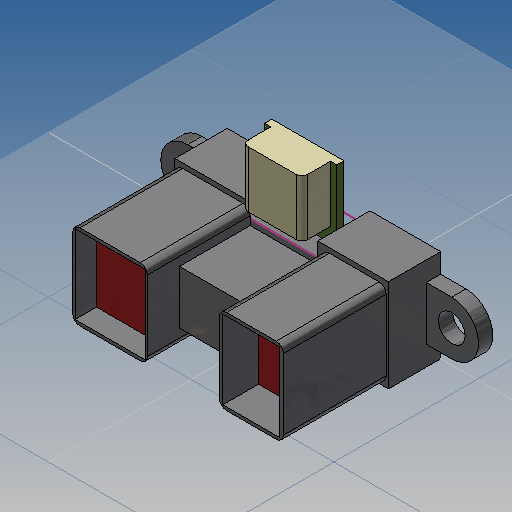
# Autodesk Inventor part: SharpDistanceRanger
Saved by Autodesk Inventor 2019 (Build 230136000, 136)
## iProperties
Created: 2013-08-17
Part Number: SharpDistanceRanger
Material: Allgemein
Document SubType Name: Modeling
Designer: Gerard
Density: 1 g/cm^3
Appearance: Vorgabe
Mass: 5.86234 g
Surface Area: 42.7278 cm^2
Volume: 5.86234 cm^3
Author: Gerard
Autodesk Inventor part; units mm, degrees
ref_plane "YZ Plane" through (0, 0, 0) normal (1, 0, 0) x (0, 1, 0)
ref_plane "XZ Plane" through (0, 0, 0) normal (0, 1, 0) x (-1, 0, 0)
ref_plane "XY Plane" through (0, 0, 0) normal (0, 0, 1) x (1, 0, 0)
sketch "Sketch1" plane through (0, 0, 0) normal (0, 0, 1) x (1, 0, 0)
  point P0 (0, 0)
sketch "Sketch2" plane through (0, 0, 0) normal (0, 0, 1) x (1, 0, 0)
  line L0 (-18.5, -6.5) -> (18.5, 6.5) construction
  line L1 (18.5, -6.5) -> (-18.5, 6.5) construction
  line L2 (-37.4614, 31.3521) -> (71.8103, 31.3521) construction
  line L3 (71.8103, 31.3521) -> (71.8103, -55.6726) construction
  line L4 (71.8103, -55.6726) -> (-37.4614, -55.6726) construction
  line L5 (-37.4614, -55.6726) -> (-37.4614, 31.3521) construction
  circle A0 centre (-18.5, 0) radius 1.875
  circle A1 centre (18.5, 0) radius 1.875
  line L6 (-14.75, 6.5) -> (14.75, 6.5)
  line L7 (14.75, 6.5) -> (14.75, -6.5)
  line L8 (14.75, -6.5) -> (-14.75, -6.5)
  line L9 (-14.75, -6.5) -> (-14.75, 6.5)
  line L10 (-14.75, 6.5) -> (14.75, -6.5) construction
  line L11 (14.75, 6.5) -> (-14.75, -6.5) construction
  circle A2 centre (-18.5, 0) radius 3.75
  circle A3 centre (18.5, 0) radius 3.75
  line L12 (-18.5, 3.75) -> (-14.75, 3.75)
  line L13 (-18.5, -3.75) -> (-14.75, -3.75)
  line L14 (18.5, 3.75) -> (14.75, 3.75)
  line L15 (18.5, -3.75) -> (14.75, -3.75)
  line L16 (-14.75, 3.75) -> (-14.75, 6.5)
  line L17 (-14.75, -3.75) -> (-14.75, -6.5)
  line L18 (14.75, 6.5) -> (14.75, 3.75)
  line L19 (14.75, -3.75) -> (14.75, -6.5)
  point P0 (0, 0)
  dimension "d0" = 37
  dimension "d1" = 13
  dimension "d30" = 3.75
  dimension "d31" = 3.75
  dimension "d32" = 29.5
  constraints: 32 end point, 5 perpendicular, 4 centre point, 4 collinear, 4 midpoint, 4 point on circle, 4 point on line, 4 tangent, 2 coincident, 2 parallel, 2 other
  measures "d0" distance of L0.start L1.start
  measures "d1" distance of L0.end L1.start
  measures "d30" diameter of A0
  measures "d31" diameter of A1
  measures "d32" distance of L6.start L6.end
extrude "Extrusion1" add sketch "Sketch2" along normal blind 2
sketch "Sketch3" plane through (0, 0, 0) normal (0, 1, 0) x (-1, 0, 0)
  line L0 (-37.7031, 80.2938) -> (71.7944, 80.2938) construction
  line L1 (71.7944, 80.2938) -> (71.7944, -6.9107) construction
  line L2 (71.7944, -6.9107) -> (-37.7031, -6.9107) construction
  line L3 (-37.7031, -6.9107) -> (-37.7031, 80.2938) construction
  line L4 (0, 0) -> (14.95, 0)
  line L5 (14.95, 0) -> (-14.95, 0)
  line L6 (-14.95, 0) -> (-14.95, 7.3126)
  line L7 (-14.95, 7.3126) -> (14.95, 7.3126)
  line L8 (14.95, 7.3126) -> (14.95, 0)
  dimension "d46" = 14.95
  dimension "d48" = 29.9
  constraints: 10 end point, 2 parallel, 2 perpendicular, 1 horizontal, 2 other
  measures "d46" distance of L4.start L4.end
  measures "d48" distance of L6.end L7.end
extrude "Extrusion2" add sketch "Sketch3" along normal mid plane 13
sketch "Sketch4" plane through (0, 0, 0) normal (0, 1, 0) x (-1, 0, 0)
  line L0 (-37.6511, 80.3124) -> (71.7381, 80.3124) construction
  line L1 (71.7381, 80.3124) -> (71.7381, -6.8059) construction
  line L2 (71.7381, -6.8059) -> (-37.6511, -6.8059) construction
  line L3 (-37.6511, -6.8059) -> (-37.6511, 80.3124) construction
  line L4 (0, 7.4343) -> (14.75, 7.4343)
  line L5 (14.75, 7.4343) -> (-14.75, 7.4343)
  line L6 (-14.75, 7.4343) -> (-14.75, 21.8343)
  line L7 (-14.75, 21.8343) -> (14.75, 21.8343)
  line L8 (14.75, 21.8343) -> (14.75, 7.4343)
  point P0 (0, 0)
  dimension "d78" = 14.75
  dimension "d79" = 29.5
  dimension "d80" = 14.4
  constraints: 10 end point, 2 parallel, 2 perpendicular, 1 horizontal, 2 other
  measures "d78" distance of L4.start L4.end
  measures "d79" distance of L6.end L7.end
  measures "d80" distance of L5.end L6.end
extrude "Extrusion3" add sketch "Sketch4" along normal mid plane 11.9
sketch "Sketch6" plane through (-14.75, 5.95, 21.8343) normal (0, 0, 1) x (1, 0, 0)
  line L0 (0, 0) -> (29.5, 0) projected
  line L1 (20.5637, -11.9) -> (8.9363, -11.9)
  line L2 (8.9363, -11.9) -> (8.9363, 0)
  line L3 (8.9363, 0) -> (20.5637, 0)
  line L4 (20.5637, 0) -> (20.5637, -11.9)
  line L5 (20.5637, -11.9) -> (8.9363, 0) construction
  line L6 (8.9363, -11.9) -> (20.5637, 0) construction
  point P0 (14.75, -5.95)
  constraints: 12 end point, 3 parallel, 2 midpoint, 1 perpendicular
extrude "Extrusion4" cut sketch "Sketch6" against normal blind 4.5
sketch "Sketch7" plane through (0, 5.95, 0) normal (0, 1, 0) x (1, 0, 0)
  line L0 (14.75, -7.4343) -> (-14.75, -7.4343) projected
  line L1 (-5.8137, -17.3343) -> (5.8137, -17.3343)
  line L2 (5.8137, -17.3343) -> (5.8137, -7.4343)
  line L3 (5.8137, -7.4343) -> (-5.8137, -7.4343)
  line L4 (-5.8137, -7.4343) -> (-5.8137, -17.3343)
  point P0 (0, 0)
  constraints: 8 end point, 2 parallel, 1 horizontal, 1 perpendicular, 1 point on line
extrude "Extrusion5" cut sketch "Sketch7" against normal blind 2.2
sketch "Sketch8" plane through (0, -5.95, 0) normal (0, -1, 0) x (1, 0, 0)
  line L0 (-14.75, 7.4343) -> (14.75, 7.4343) projected
  line L1 (-5.8137, 17.3343) -> (5.8137, 17.3343)
  line L2 (5.8137, 17.3343) -> (5.8137, 7.4343)
  line L3 (5.8137, 7.4343) -> (-5.8137, 7.4343)
  line L4 (-5.8137, 7.4343) -> (-5.8137, 17.3343)
  point P0 (0, 0)
  constraints: 8 end point, 2 parallel, 1 horizontal, 1 perpendicular, 1 point on line
extrude "Extrusion6" cut sketch "Sketch8" against normal blind 2.2
sketch "Sketch9" plane through (-5.8137, -5.95, 21.8343) normal (1, 0, 0) x (0, 0, -1)
  line L0 (0, 0) -> (0, 11.9) projected
  line L1 (14.4, 0) -> (0, 0) projected
  line L2 (14.4, 2.2) -> (14.4, 0) projected
  line L3 (14.4, 2.2) -> (4.5, 2.2) projected
  line L4 (4.5, 2.2) -> (4.5, 9.7) projected
  line L5 (4.5, 9.7) -> (14.4, 9.7) projected
  line L6 (14.4, 11.9) -> (14.4, 9.7) projected
  line L7 (0, 11.9) -> (14.4, 11.9) projected
  point P0 (21.8343, 5.95)
extrude "Extrusion7" add sketch "Sketch9" along normal blind 1.514
sketch "Sketch10" plane through (5.8137, -5.95, 21.8343) normal (-1, 0, 0) x (0, 0, 1)
  line L0 (0, 11.9) -> (0, 0) projected
  line L1 (-14.4, 11.9) -> (0, 11.9) projected
  line L2 (-14.4, 9.7) -> (-14.4, 11.9) projected
  line L3 (-14.4, 9.7) -> (-4.5, 9.7) projected
  line L4 (-4.5, 9.7) -> (-4.5, 2.2) projected
  line L5 (-4.5, 2.2) -> (-14.4, 2.2) projected
  line L6 (-14.4, 0) -> (-14.4, 2.2) projected
  line L7 (0, 0) -> (-14.4, 0) projected
  point P0 (-21.8343, 5.95)
extrude "Extrusion8" add sketch "Sketch10" along normal blind 0.014
sketch "Sketch11" plane through (-14.75, -5.95, 21.8343) normal (0, 0, 1) x (1, 0, 0)
  line L0 (0, 11.9) -> (10.4503, 11.9) projected
  line L1 (0.3252, 11.45) -> (10.1252, 11.45)
  line L2 (10.1252, 11.45) -> (10.1252, 0.45)
  line L3 (10.1252, 0.45) -> (0.3252, 0.45)
  line L4 (0.3252, 0.45) -> (0.3252, 11.45)
  line L5 (0.3252, 11.45) -> (10.1252, 0.45) construction
  line L6 (10.1252, 11.45) -> (0.3252, 0.45) construction
  point P0 (14.75, 5.95)
  point P1 (5.2252, 5.95)
  dimension "d134" = 9.8
  dimension "d135" = 11
  constraints: 12 end point, 3 parallel, 2 midpoint, 1 perpendicular
  measures "d134" distance of L1.start L1.end
  measures "d135" distance of L1.end L2.end
extrude "Extrusion9" cut sketch "Sketch11" against normal blind 3
sketch "Sketch12" plane through (14.75, -5.95, 21.8343) normal (0, 0, 1) x (1, 0, 0)
  line L0 (0, 0) -> (-8.9503, 0) projected
  line L1 (-8.4752, 11.45) -> (-0.4752, 11.45)
  line L2 (-0.4752, 11.45) -> (-0.4752, 0.45)
  line L3 (-0.4752, 0.45) -> (-8.4752, 0.45)
  line L4 (-8.4752, 0.45) -> (-8.4752, 11.45)
  line L5 (-8.4752, 11.45) -> (-0.4752, 0.45) construction
  line L6 (-0.4752, 11.45) -> (-8.4752, 0.45) construction
  point P0 (-14.75, 5.95)
  point P1 (-4.4752, 5.95)
  dimension "d138" = 8
  dimension "d139" = 11
  constraints: 12 end point, 3 parallel, 2 midpoint, 1 perpendicular
  measures "d138" distance of L1.start L1.end
  measures "d139" distance of L1.end L2.end
extrude "Extrusion10" cut sketch "Sketch12" against normal blind 5
sketch "Sketch13" plane through (-14.95, 6.5, 0) normal (0, 1, 0) x (1, 0, 0)
  line L0 (29.9, 0) -> (0, 0) projected
  line L1 (0, -7.3126) -> (29.9, -7.3126) projected
  line L2 (14.95, 0) -> (9.9, 0)
  line L3 (9.9, 0) -> (20, 0)
  line L4 (20, 0) -> (20, -7.3126)
  line L5 (20, -7.3126) -> (9.9, -7.3126)
  line L6 (9.9, -7.3126) -> (9.9, 0)
  line L7 (20, 0) -> (9.9, 0)
  line L8 (9.9, 0) -> (9.9, -1)
  line L9 (9.9, -1) -> (20, -1)
  line L10 (20, -1) -> (20, 0)
  dimension "d142" = 5.05
  dimension "d143" = 10.1
  dimension "d144" = 1
  constraints: 18 end point, 4 parallel, 3 point on line, 2 horizontal, 2 perpendicular
  measures "d142" distance of L2.start L2.end
  measures "d143" distance of L4.end L5.end
  measures "d144" distance of L8.end L7.end
extrude "Extrusion11" cut sketch "Sketch13" against normal blind 2
sketch "Sketch14" plane through (-14.95, 4.5, 0) normal (0, 1, 0) x (1, 0, 0)
  line L0 (9.9, -7.3126) -> (9.9, 0) projected
  line L1 (20, -7.3126) -> (9.9, -7.3126) projected
  line L2 (20, 0) -> (20, -7.3126) projected
  line L3 (9.9, 0) -> (20, 0) projected
  point P0 (14.95, 0)
sketch "Sketch15" plane through (-14.95, 4.5, 0) normal (0, 1, 0) x (1, 0, 0)
  line L0 (9.9, -7.3126) -> (9.9, 0) projected
  line L1 (20, 0) -> (20, -7.3126) projected
  line L2 (20, -3.6563) -> (9.9, -3.6563)
  line L3 (9.9, -3.6563) -> (9.9, -4.6563)
  line L4 (9.9, -4.6563) -> (20, -4.6563)
  line L5 (20, -4.6563) -> (20, -3.6563)
  point P0 (14.95, 0)
  dimension "d147" = 1
  constraints: 8 end point, 2 parallel, 1 horizontal, 1 midpoint, 1 perpendicular, 1 point on line
  measures "d147" distance of L3.end L2.end
extrude "Extrusion12" add sketch "Sketch15" along normal blind 9.9
sketch "Sketch16" plane through (0, 0, 0) normal (0, 0, -1) x (-1, 0, 0)
  line L0 (-14.95, 6.5) -> (-5.05, 6.5) projected
  line L1 (-14.5, 6) -> (14.5, 6)
  line L2 (14.5, 6) -> (14.5, -6)
  line L3 (14.5, -6) -> (-14.5, -6)
  line L4 (-14.5, -6) -> (-14.5, 6)
  line L5 (-14.5, 6) -> (14.5, -6) construction
  line L6 (14.5, 6) -> (-14.5, -6) construction
  point P0 (0, 0)
  dimension "d150" = 29
  dimension "d151" = 12
  constraints: 12 end point, 3 parallel, 2 midpoint, 1 perpendicular
  measures "d150" distance of L1.start L1.end
  measures "d151" distance of L1.end L2.end
extrude "Extrusion13" cut sketch "Sketch16" against normal blind 2
sketch "Sketch17" plane through (-5.05, 4.5, 4.6563) normal (0, 0, 1) x (1, 0, 0)
  line L0 (10.1, 0) -> (0, 0) projected
  line L1 (0.876, 2) -> (9.224, 2)
  line L2 (9.224, 2) -> (9.224, 9.9)
  line L3 (9.224, 9.9) -> (0.876, 9.9)
  line L4 (0.876, 9.9) -> (0.876, 2)
  line L5 (0.876, 2) -> (9.224, 9.9) construction
  line L6 (9.224, 2) -> (0.876, 9.9) construction
  point P0 (5.05, -4.5)
  point P1 (5.05, 5.95)
  constraints: 12 end point, 3 parallel, 2 midpoint, 1 perpendicular
extrude "Extrusion14" add sketch "Sketch17" along normal blind 4
sketch "Sketch18" plane through (-14.95, 4.5, 0) normal (0, 1, 0) x (1, 0, 0)
  line L0 (20, -2) -> (9.9, -2) projected
  line L1 (9.9, -3.6563) -> (9.9, -2) projected
  line L2 (9.9, -3.6563) -> (20, -3.6563) projected
  line L3 (20, -2) -> (20, -3.6563) projected
  point P0 (14.95, 0)
sketch "Sketch19" plane through (-14.95, 4.5, 0) normal (0, 1, 0) x (1, 0, 0)
  line L0 (9.9, -3.6563) -> (20, -3.6563) projected
  line L1 (11.95, -4.4845) -> (17.95, -4.4845)
  line L2 (17.95, -4.4845) -> (17.95, -2.8282)
  line L3 (17.95, -2.8282) -> (11.95, -2.8282)
  line L4 (11.95, -2.8282) -> (11.95, -4.4845)
  line L5 (11.95, -4.4845) -> (17.95, -2.8282) construction
  line L6 (17.95, -4.4845) -> (11.95, -2.8282) construction
  point P0 (14.95, 0)
  point P1 (14.95, -3.6563)
  dimension "d156" = 6
  constraints: 12 end point, 3 midpoint, 2 parallel, 1 perpendicular
  measures "d156" distance of L1.start L1.end
extrude "Extrusion15" add sketch "Sketch19" along normal blind 7
fillet "Fillet1" radius 0.8 2 edges at (4.174, 10.45, 8.6563) (-4.174, 10.45, 8.6563)
fillet "Fillet2" radius 1 8 edges at (14.75, 5.95, 14.6343) (14.75, -5.95, 14.6343) (-14.75, 5.95, 14.6343) (-4.2997, 5.95, 14.6343) (5.7997, 5.95, 14.6343) (5.7997, -5.95, 14.6343) (-4.2997, -5.95, 14.6343) (-14.75, -5.95, 14.6343)
body "Solid1"
